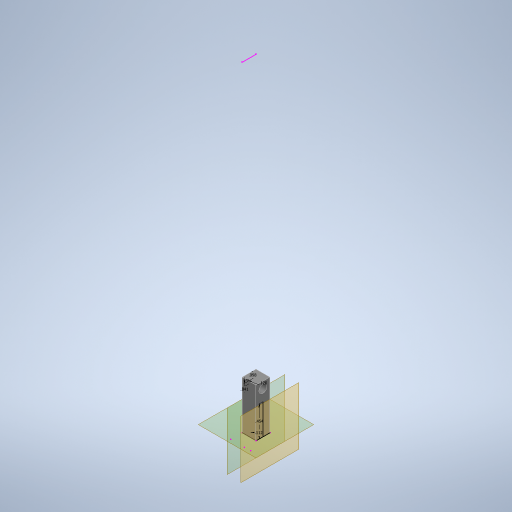
# Autodesk Inventor part: rod1
Saved by Autodesk Inventor 2024 (Build 280153000, 153)
## iProperties
Created: 2023-04-14
Part Number: rod1
Material: Generic
Document SubType Name: Modeling
Designer: Fujitsu
Density: 1 g/cm^3
Appearance: Default
Author: Fujitsu
Autodesk Inventor part; units mm, degrees
ref_plane "YZ Plane" through (0, 0, 0) normal (1, 0, 0) x (0, 1, 0)
ref_plane "XZ Plane" through (0, 0, 0) normal (0, 1, 0) x (-1, 0, 0)
ref_plane "XY Plane" through (0, 0, 0) normal (0, 0, 1) x (1, 0, 0)
ref_plane "Work Plane2" through (-2.3036, 0, -9.6783) normal (1, 0, 0) x (0, 0, -1)
sketch "Sketch1" plane through (-2.3036, 0, -9.6783) normal (1, 0, 0) x (0, 0, -1)
  line L0 (0, 0) -> (-5.2832, 0) projected
  line L1 (-2.6416, 0) -> (-2.6416, 10.3378)
  line L2 (-2.6416, 10.3378) -> (-2.6416, 11.1315)
  line L3 (-2.6416, 0) -> (-2.6416, 11.5316)
  point P0 (-9.6783, 0)
  dimension "d24" = 11.5316
  constraints: 6 end point, 3 vertical, 1 midpoint
  measures "d24" distance of L1.start L3.end
ref_plane "Work Plane1" through (-2.3036, 0, -9.6783) normal (1, 0, 0) x (0, 0, -1)
sketch "Sketch2" plane through (-2.3036, 0, -9.6783) normal (1, 0, 0) x (0, 0, -1)
  point P0 (-9.6783, 0)
ref_plane "Work Plane3" through (-2.3036, 0, -9.6783) normal (1, 0, 0) x (0, 0, -1)
ref_plane "Work Plane6" through (-7.5868, 0, -9.6783) normal (-1, 0, 0) x (0, 0, 1)
sketch "Sketch5" plane through (-7.5868, 0, -9.6783) normal (-1, 0, 0) x (0, 0, 1)
  line L0 (5.2832, 122.2682) -> (0, 122.2682) projected
  line L1 (0, 0) -> (5.2832, 0) projected
  line L2 (2.6416, 0) -> (2.6416, 14.7688)
  line L3 (2.6416, 14.7688) -> (2.6416, 15.7975)
  line L4 (2.6416, 15.7975) -> (2.6416, 18.2867)
  circle A0 centre (2.6416, 15.7975) radius 1.524
  point P0 (9.6783, 0)
  dimension "d25" = 1.0287
  dimension "d26" = 2.4892
  dimension "d27" = 3.048
  constraints: 6 end point, 2 coincident, 2 vertical, 1 centre point, 1 midpoint
  measures "d25" distance of L2.end L3.end
  measures "d26" distance of L3.end L4.end
  measures "d27" diameter of A0
hole "Hole3" [suppressed]
ref_plane "Work Plane5" through (-7.5868, 0, -9.6783) normal (0, -1, 0) x (1, 0, 0)
sketch "Sketch6" plane through (-7.5868, 0, -9.6783) normal (0, -1, 0) x (1, 0, 0)
  line L0 (0, 0) -> (0, 5.2832) projected
  line L1 (5.2832, 0) -> (0, 0) projected
  line L2 (0, 5.2832) -> (5.2832, 5.2832)
  line L3 (5.2832, 5.2832) -> (5.2832, 0)
  line L4 (5.2832, 0) -> (0, 0)
  line L5 (0, 0) -> (0, 5.2832)
  arc A0 (3.5677, 2.2318) -> (3.582, 3.0171) centre (2.6416, 2.6416) ccw projected
  circle A1 centre (2.6416, 2.6416) radius 1.4224
  point P0 (7.5868, 9.6783)
  dimension "d35" = 2.8448
  constraints: 8 end point, 2 parallel, 1 centre point, 1 coincident, 1 horizontal, 1 perpendicular
  measures "d35" diameter of A1
extrude "Extrusion3" add sketch "Sketch6" against normal blind 18.288 contours L0 L2 L3 L1 | A1
hole "Hole4" at (-7.5868, 15.7975, -7.0367) direction (1, 0, 0) diameter 3.048 end through all
extrude "Extrusion4" cut sketch "Sketch6" against normal blind 11.684 contours A1
thread "Thread1" size "4-40 UNC" class "2B" standard "ANSI Unified Screw Threads" full length
body "Solid1"
